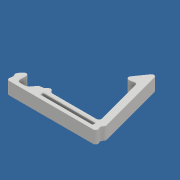
# Autodesk Inventor part: smaho_mount
Saved by Autodesk Inventor 2017 (Build 210142000, 142)
## iProperties
Part Number: smaho_mount
Material: 一般
Document SubType Name: Modeling
Designer: uhiit
Density: 1 g/cm^3
Appearance: 既定
Mass: 11.1879 g
Surface Area: 68.3105 cm^2
Volume: 11.1879 cm^3
Author: uhiit
Autodesk Inventor part; units mm, degrees
ref_plane "YZ Plane" through (0, 0, 0) normal (1, 0, 0) x (0, 1, 0)
ref_plane "XZ Plane" through (0, 0, 0) normal (0, 1, 0) x (-1, 0, 0)
ref_plane "XY Plane" through (0, 0, 0) normal (0, 0, 1) x (1, 0, 0)
sketch "スケッチ1" plane through (0, 0, 0) normal (0, 0, 1) x (1, 0, 0)
  line L0 (0, 0) -> (50, 0)
  line L1 (7.5, 13) -> (7.5, 3)
  circle A0 centre (12.5, 8) radius 5 construction
  line L2 (17.5, 3) -> (17.5, 8) construction
  line L3 (7.5, 3) -> (15.2999, 3.0285)
  line L4 (15.2999, 3.0285) -> (58.3182, 64.465)
  line L5 (15.2999, 3.0285) -> (17.5, 3.0285) construction
  ellipse E0 centre (7.5, 0) end of major axis (0, 0) minor radius 13 (14.7939, 3.0267) -> (14.7936, 3.0285) ccw
  ellipse E1 centre (7.5, 0) end of major axis (0, 0) minor radius 13 (7.5, 13) -> (0, 0) ccw
  line L6 (58.3182, 64.465) -> (75.5915, 0)
  line L7 (58.3182, 64.465) -> (125.0572, 64.465) construction
  line L8 (75.5915, 0) -> (50, 0)
  dimension "d0" = 50
  dimension "d1" = 13
  dimension "d2" = 7.5
  dimension "d3" = 10
  dimension "d4" = 5
  dimension "d5" = 8
  dimension "d6" = 7.8
  dimension "d7" = 75
  dimension "d8" = 55
  dimension "d9" = 75
  constraints: 18 end point, 5 horizontal, 4 point on line, 1 coincident, 1 collinear, 1 equal length, 1 horizontal alignment, 1 perpendicular, 1 vertical, 10 other
  measures "d0" distance of L0.start L0.end
  measures "d1" distance from line of L1.start L0
  measures "d2" horizontal distance of L1.start L0.start
  measures "d3" distance of L1.start L1.end
  measures "d4" distance from line of L1 point (12.5, 8)
  measures "d5" distance from line of L0 point (12.5, 8)
  measures "d6" distance of L1.end L3.end
  measures "d7" distance of L3.end L4.end
  measures "d8" angle of L5 L4
  measures "d9" angle of L6 L7
extrude "押し出し1" add sketch "スケッチ1" along normal blind 10
sketch "スケッチ2" plane through (0, 0, 10) normal (0, 0, 1) x (1, 0, 0)
  line L0 (75.5915, 0) -> (58.3182, 64.465) projected
  line L1 (74.78, 3.0285) -> (58.3182, 64.465)
  line L2 (58.3182, 64.465) -> (15.2999, 3.0285) projected
  line L3 (58.3182, 64.465) -> (15.2999, 3.0285)
  line L4 (74.78, 3.0285) -> (15.2999, 3.0285)
  line L5 (25.8653, 8.5285) -> (56.0583, 51.6486)
  line L6 (56.0583, 51.6486) -> (67.6123, 8.5285)
  line L7 (67.6123, 8.5285) -> (25.8653, 8.5285)
  point P0 (0, 0)
  dimension "d12" = 5.5
  constraints: 12 end point, 2 collinear, 1 horizontal, 2 other
  measures "d12" distance between parallel lines of L4 L7
extrude "押し出し2" cut sketch "スケッチ2" against normal blind 10 contours L5 L6 L7
sketch "スケッチ3" plane through (0, 0, 10) normal (0, 0, 1) x (1, 0, 0)
  line L0 (67.5, 3) -> (26, 3)
  line L1 (26, 3) -> (26, 5.2)
  line L2 (26, 5.2) -> (67.5, 5.2)
  line L3 (67.5, 5.2) -> (67.5, 3)
  point P0 (0, 0)
  point P1 (26, 3)
  dimension "d15" = 26
  dimension "d16" = 3
  dimension "d17" = 41.5
  dimension "d18" = 2.2
  dimension "d19" = 41.5
  constraints: 8 end point, 2 parallel, 1 horizontal, 1 perpendicular
  measures "d15" horizontal distance of point (0, 0) point (26, 3)
  measures "d16" vertical distance of point (0, 0) point (26, 3)
  measures "d17" distance of point (26, 3) L0.start
  measures "d18" distance of L0.end L1.end
  measures "d19" distance of L0.start L0.end
extrude "押し出し3" cut sketch "スケッチ3" against normal blind 10
fillet "フィレット1" radius 2 7 edges at (58.3182, 64.465, 5) (56.0583, 51.6486, 5) (25.8653, 8.5285, 5) (67.6123, 8.5285, 5) (75.5915, 0, 5) (0, 0, 5) (7.5, 13, 5)
fillet "フィレット2" radius 2 1 edges at (7.5, 3, 5)
fillet "フィレット3" radius 4.5 1 edges at (15.2999, 3.0285, 5)
sketch "スケッチ5" plane through (0, 0, 10) normal (0, 0, 1) x (1, 0, 0)
  arc A0 (28.069, 11.6757) -> (29.7073, 8.5285) centre (29.7073, 10.5285) ccw projected
  ellipse E0 centre (7.5, 0) end of major axis (7.5, -13) minor radius 7.5 (4.2074, 11.6803) -> (0.1079, 2.1969) ccw projected
  line L0 (1.3247, 7.3775) -> (2.4858, 5.1177)
  line L1 (2.4858, 5.1177) -> (2.3363, 2.6665)
  line L2 (2.3363, 2.6665) -> (0.5732, 0.7059)
  arc A1 (0.1079, 2.1969) -> (2.0982, 0) centre (2.0982, 2) ccw projected
  line L3 (28.069, 11.6757) -> (25.4208, 11.2334)
  line L4 (25.4208, 11.2334) -> (23.9255, 10.1018)
  line L5 (23.9255, 10.1018) -> (22.9593, 9.0274)
  line L6 (22.9593, 9.0274) -> (20.4102, 8.6016)
  line L7 (20.4102, 8.6016) -> (20.4102, 8.6016)
  line L8 (20.4102, 8.6016) -> (19.1511, 8.5285)
  line L9 (55.8581, 60.9516) -> (16.6376, 4.9389) projected
  arc A2 (72.9851, 0) -> (74.9169, 2.5176) centre (72.9851, 2) ccw projected
  line L10 (74.6592, 0.9058) -> (71.437, 4.2683)
  line L11 (71.437, 4.2683) -> (73.6147, 7.3775)
  line L12 (74.9169, 2.5176) -> (59.4283, 60.3221) projected
  line L13 (57.1684, 47.5057) -> (66.9377, 11.0462) projected
  line L14 (58.5658, 42.2904) -> (57.1684, 47.5057)
  arc A3 (57.1684, 47.5057) -> (53.5982, 48.1352) centre (55.2365, 46.988) ccw projected
  line L15 (53.9799, 48.544) -> (51.0657, 48.2348)
  line L16 (51.0657, 48.2348) -> (47.1702, 48.544)
  line L17 (28.069, 11.6757) -> (53.5982, 48.1352)
  line L18 (47.1702, 48.544) -> (19.1511, 8.5285)
  arc A4 (7.5, 10.1541) -> (4.2074, 11.6803) centre (5.5, 10.1541) ccw projected
  ellipse E1 centre (7.5, 0) end of major axis (7.5, -13) minor radius 7.5 (4.2074, 11.6803) -> (0.1079, 2.1969) ccw projected
  arc A5 (0.1079, 2.1969) -> (2.0982, 0) centre (2.0982, 2) ccw projected
  line L19 (2.0982, 0) -> (72.9851, 0) projected
  arc A6 (72.9851, 0) -> (74.9169, 2.5176) centre (72.9851, 2) ccw projected
  line L20 (74.9169, 2.5176) -> (59.4283, 60.3221) projected
  arc A7 (59.4283, 60.3221) -> (55.8581, 60.9516) centre (57.4964, 59.8044) ccw projected
  line L21 (55.8581, 60.9516) -> (16.6376, 4.9389) projected
  arc A8 (12.9679, 3.02) -> (16.6376, 4.9389) centre (12.9514, 7.52) ccw projected
  line L22 (12.9679, 3.02) -> (9.5073, 3.0073) projected
  arc A9 (7.5, 5.0073) -> (9.5073, 3.0073) centre (9.5, 5.0073) ccw projected
  line L23 (7.5, 5.0073) -> (7.5, 10.1541) projected
  line L24 (67.5, 5.2) -> (67.5, 3) projected
  line L25 (67.5, 3) -> (26, 3) projected
  line L26 (26, 3) -> (26, 5.2) projected
  line L27 (26, 5.2) -> (67.5, 5.2) projected
  line L28 (65.0058, 8.5285) -> (29.7073, 8.5285) projected
  arc A10 (28.069, 11.6757) -> (29.7073, 8.5285) centre (29.7073, 10.5285) ccw projected
  line L29 (28.069, 11.6757) -> (53.5982, 48.1352) projected
  arc A11 (57.1684, 47.5057) -> (53.5982, 48.1352) centre (55.2365, 46.988) ccw projected
  line L30 (57.1684, 47.5057) -> (66.9377, 11.0462) projected
  arc A12 (65.0058, 8.5285) -> (66.9377, 11.0462) centre (65.0058, 10.5285) ccw projected
  line L31 (1.3247, 7.3775) -> (-3.2011, 4.1)
  line L32 (-3.2011, 4.1) -> (-1.2016, -1.2678)
  line L33 (-1.2016, -1.2678) -> (0.616, 0.6572)
  line L34 (73.6147, 7.3775) -> (77.245, 2.5176)
  line L35 (77.245, 2.5176) -> (79.5635, 0.8938)
  line L36 (79.5635, 0.8938) -> (74.5718, 0.7825)
  point P0 (0, 0)
  constraints: 44 end point, 5 point on circle, 4 point on line, 2 parallel, 1 collinear, 3 other
extrude "押し出し4" cut sketch "スケッチ5" against normal blind 10 contours L3 L4 L5 L6 L8 L9 L16 L15 A3 L17 | L12 A2 L10 L11 | L0 L1 L2 A1 E0
fillet "フィレット4" radius 2 14 edges at (74.6592, 0.9058, 5) (71.437, 4.2683, 5) (73.6147, 7.3775, 5) (28.069, 11.6757, 5) (23.9255, 10.1018, 5) (22.9593, 9.0274, 5) (19.1511, 8.5285, 5) (53.9799, 48.544, 5) (47.1702, 48.544, 5) (51.0657, 48.2348, 5) (1.3247, 7.3775, 5) (2.4858, 5.1177, 5) (2.3363, 2.6665, 5) (0.5732, 0.7059, 5)
